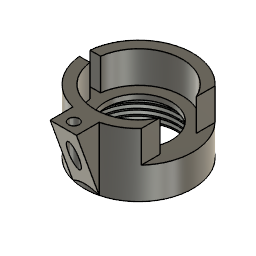
Lenshouder schroefdraad + Mount (Autodesk Fusion 360 design; units mm, degrees)
part number: 2026-06-04-13-28-36-774
Autodesk Fusion 360 part; units mm, degrees
note: some values were not read from the file. Chosen so that the rebuilt part matches the saved one: which face or edge a step refers to.
sketch "Sketch2" plane through (0, 0, 0) normal (0, 0, 1) x (1, 0, 0)
  circle A0 centre (0, 0) radius 15
  dimension "d8" = 30
  constraint coincident A0.centre origin
  measures "d8" diameter of A0
extrude "Extrude3" add sketch "Sketch2" along normal blind 10 thin wall 5.5 outside makes body 1
sketch "Sketch1" plane through (0, 0, 10) normal (0, 0, 1) x (1, 0, 0)
  circle A0 centre (0, 0) radius 16.5
  circle A1 centre (0, 0) radius 15
  circle A2 centre (0, 0) radius 20.5
  dimension "d1" = 33
  constraint coincident A0.centre A1.centre
  measures "d1" diameter of A0
extrude "Extrude1" add sketch "Sketch1" along normal blind 14 thin wall 4 outside separate body contours A0 | A1 makes body 2
extrude "Extrude2" add sketch "Sketch1" along normal blind 2 thin wall 4 inside contours A0 | A1 bodies 2
sketch "Sketch3" plane through (0, 0, 24) normal (0, 0, 1) x (-1, 0, 0)
  circle A0 centre (0, 0) radius 16.5
  circle A1 centre (0, 0) radius 20.5
  line L0 (-21, 20) -> (-15, 20)
  line L1 (-15, 20) -> (-15, -20)
  line L2 (-15, -20) -> (-21, -20)
  line L3 (-21, -20) -> (-21, 20)
  line L4 (-21, 20) -> (-15, -20) construction
  line L5 (-15, 20) -> (-21, -20) construction
  line L6 (15.5, 2) -> (21.5, 2)
  line L7 (21.5, 2) -> (21.5, -2)
  line L8 (21.5, -2) -> (15.5, -2)
  line L9 (15.5, -2) -> (15.5, 2)
  line L10 (15.5, 2) -> (21.5, -2) construction
  line L11 (21.5, 2) -> (15.5, -2) construction
  point P0 (-18, 0)
  point P1 (18.5, 0)
  dimension "d12" = 6
  dimension "d13" = 40
  dimension "d16" = 15
  dimension "d17" = 20
  dimension "d18" = 6
  dimension "d19" = 4
  dimension "d20" = 15.5
  dimension "d21" = 2
  constraint horizontal L0
  constraint perpendicular L0 L1
  constraint parallel L0 L2
  constraint parallel L1 L3
  constraint coincident L4 P0
  constraint coincident L5 P0
  constraint horizontal L6
  constraint perpendicular L6 L7
  constraint parallel L6 L8
  constraint parallel L7 L9
  constraint coincident L10 P1
  constraint coincident L11 P1
  measures "d12" distance of L1.end L2.end
  measures "d13" distance of L0.end L1.end
  measures "d16" distance of A0.centre L1
  measures "d17" distance of A0.centre L2
  measures "d18" distance of L7.end L8.end
  measures "d19" distance of L6.end L7.end
  measures "d20" distance of A0.centre L9
  measures "d21" distance of A0.centre L8
extrude "Extrude4" cut sketch "Sketch3" against normal blind 12 contours A0 A1 L6 L8 | A0 A1 L1 bodies 2
thread "Thread1" "ISO Metric profile 32.0 M32x2 M32x2 6H" major diameter 32.2565 minor diameter 30.0224 pitch 2 angle 60 modelled right hand crest width 0.5434 on face at (14.9814, -0.7477, 6.6667) crest through (15.0112, 0, 0.5) on bodies 1
combine "Combine1" operation add target body 2 tool bodies 1
sketch "Top Taper profile" plane through (0, 0, 24) normal (0, 0, 1) x (-1, 0, 0)
  line L0 (-15, 13.9732) -> (-15, 6.8739)
  arc A0 (16.3783, 2) -> (-15, 6.8739) centre (0, 0) ccw
  line L1 (16.3783, 2) -> (20.4022, 2)
  arc A1 (20.4022, 2) -> (-15, 13.9732) centre (0, 0) ccw
  line L2 (-5, 28.5) -> (5, 28.5)
  line L3 (5, 28.5) -> (5, 16.5)
  line L4 (5, 16.5) -> (-5, 16.5)
  line L5 (-5, 16.5) -> (-5, 28.5)
  line L6 (-5, 28.5) -> (5, 16.5) construction
  line L7 (5, 28.5) -> (-5, 16.5) construction
  circle A2 centre (0, 0) radius 12.5
  line L8 (0, -1.75) -> (0, -22.5)
  point P0 (0, 22.5)
  dimension "d26" = 10
  dimension "d27" = 12
  constraint horizontal L2
  constraint perpendicular L2 L3
  constraint parallel L2 L4
  constraint parallel L3 L5
  constraint coincident L6 P0
  constraint coincident L7 P0
  constraint coincident P0 L8
  constraint tangent A0 L4
  measures "d26" distance of L3.end L4.end
  measures "d27" distance of L2.end L3.end
sketch "Lower taper profile" plane through (0, 0, 0) normal (0, 0, -1) x (1, 0, 0)
  spline S0 degree 3 poles (-4.1754, -15.5784) (-6.17, -14.97) (-8.0275, -13.9804) (-11.2341, -11.3583) (-12.5588, -9.7593) (-14.5032, -6.1653) (-15.1133, -4.21) (-15.5416, -0.2024) (-15.3662, 1.81) (-14.4742, 4.8781) (-14.0074, 5.9816) (-12.8291, 8.0472) (-12.1238, 9.0032) (-11.3134, 9.8662) knots 0 0 0 0 0.625605 0.625605 1.243004 1.243004 1.852196 1.852196 2.453177 2.453177 2.811837 2.811837 3.167466 3.167466 3.167466 3.167466
  arc A0 (11.3134, 9.8662) -> (-11.3134, 9.8662) centre (0, 0) ccw
  spline S1 degree 3 poles (11.3134, 9.8662) (12.6598, 8.4322) (13.7111, 6.7474) (15.1237, 3.045) (15.4614, 1.0595) (15.3612, -2.9578) (14.9137, -4.9505) (13.2734, -8.6802) (12.0868, -10.3769) (9.7087, -12.6691) (8.7081, -13.428) (6.5416, -14.7018) (5.3822, -15.2103) (4.1754, -15.5784) knots 0 0 0 0 0.590122 0.590122 1.188445 1.188445 1.794967 1.794967 2.409684 2.409684 2.784681 2.784681 3.162702 3.162702 3.162702 3.162702
  arc A1 (-4.1754, -15.5784) -> (4.1754, -15.5784) centre (0, 0) ccw
  circle A2 centre (0, 0) radius 20.5
  line L0 (5, 19.8809) -> (-5, 19.8809)
  line L1 (-5, 19.8809) -> (-5, 15.0112)
  line L2 (-5, 15.0112) -> (5, 15.0112)
  line L3 (5, 15.0112) -> (5, 19.8809)
  line L4 (5, 19.8809) -> (-5, 15.0112) construction
  line L5 (-5, 19.8809) -> (5, 15.0112) construction
  point P0 (0, 17.446)
  dimension "d28" = 10
  constraint horizontal L0
  constraint perpendicular L0 L1
  constraint parallel L0 L2
  constraint parallel L1 L3
  constraint coincident L4 P0
  constraint coincident L5 P0
  constraint tangent A0 L2
  constraint coincident A2 L0.end
  constraint coincident A2 L0.start
  measures "d28" distance of L1.end L2.end
loft "Loft1" add profiles "Top Taper profile", "Lower taper profile" section 1 contours A1 L2 L3 L5 section 2 contours L0 L1 L2 L3 bodies 2
sketch "Sketch6" plane through (0, 0, 24) normal (0, 0, 1) x (-1, 0, 0)
  line L0 (-15, 13.9732) -> (-15, 6.8739)
  arc A0 (16.3783, 2) -> (-15, 6.8739) centre (0, 0) ccw
  line L1 (16.3783, 2) -> (20.4022, 2)
  arc A1 (20.4022, 2) -> (5, 19.8809) centre (0, 0) ccw
  line L2 (5, 19.8809) -> (5, 28.5)
  line L3 (5, 28.5) -> (-5, 28.5)
  line L4 (-5, 28.5) -> (-5, 19.8809)
  arc A2 (-5, 19.8809) -> (-15, 13.9732) centre (0, 0) ccw
  circle A3 centre (0, 24.5) radius 2
  line L5 (0, -1.75) -> (0, -22.5)
  dimension "d29" = 4
  dimension "d30" = 4
  constraint coincident A3.centre L5
  measures "d29" diameter of A3
  measures "d30" distance of L3 A3.centre
extrude "Extrude5" cut sketch "Sketch6" along normal through all and the other way through all contours A3 bodies 2
scale "Scale2" factor 1.008 about (-20.5, 0, 0) bodies 2
